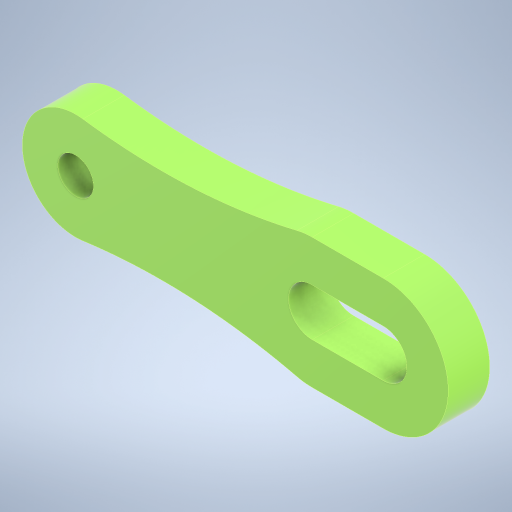
# Autodesk Inventor part: Elbow holder
Saved by Autodesk Inventor 2023 (Build 270158000, 158)
## iProperties
Created: 2022-05-02
Part Number: Elbow holder
Material: Phenolic Resin
Document SubType Name: Modeling
Designer: Devin
Density: 1.38 g/cm^3
Appearance: Light Green
Author: Devin
Autodesk Inventor part; units mm, degrees
ref_plane "YZ Plane" through (0, 0, 0) normal (1, 0, 0) x (0, 1, 0)
ref_plane "XZ Plane" through (0, 0, 0) normal (0, 1, 0) x (-1, 0, 0)
ref_plane "XY Plane" through (0, 0, 0) normal (0, 0, 1) x (1, 0, 0)
sketch "Sketch1" plane through (0, 0, 0) normal (0, 0, 1) x (1, 0, 0)
  line L0 (1.016, 0) -> (4.064, 0)
  line L1 (5.08, -1.016) -> (5.08, -1.016)
  line L2 (4.064, -2.032) -> (1.016, -2.032)
  line L3 (0, -1.016) -> (0, -1.016)
  line L4 (1.016, -3.81) -> (4.064, -3.81)
  line L5 (6.858, -1.016) -> (6.858, -1.016)
  line L6 (4.064, 1.778) -> (1.016, 1.778)
  line L7 (-1.778, -1.016) -> (-1.778, -1.016)
  arc A0 (6.858, -1.016) -> (4.064, 1.778) centre (4.064, -1.016) ccw
  arc A1 (4.064, -3.81) -> (6.858, -1.016) centre (4.064, -1.016) ccw
  arc A2 (5.08, -1.016) -> (4.064, 0) centre (4.064, -1.016) ccw
  arc A3 (4.064, -2.032) -> (5.08, -1.016) centre (4.064, -1.016) ccw
  arc A4 (1.016, 0) -> (0, -1.016) centre (1.016, -1.016) ccw
  arc A5 (0, -1.016) -> (1.016, -2.032) centre (1.016, -1.016) ccw
  circle A6 centre (-9.144, -1.016) radius 2.286
  circle A7 centre (-9.144, -1.016) radius 0.762
  arc A8 (1.016, 1.778) -> (-1.778, -1.016) centre (1.016, -1.016) ccw
  arc A9 (-1.778, -1.016) -> (1.016, -3.81) centre (1.016, -1.016) ccw
  arc A10 (-8.8323, 1.2486) -> (0.3651, 1.7011) centre (-5.4362, 25.9197) ccw
  arc A11 (0.3651, -3.7331) -> (-8.8323, -3.2806) centre (-5.4362, -27.9517) ccw
  line L8 (-8.0967, 1.016) -> (-0.9017, 1.016) construction
  line L9 (-8.0967, -3.048) -> (-0.9017, -3.048) construction
  line L10 (-6.858, -1.016) -> (-1.778, -1.016) construction
  point P0 (0, 0)
  point P1 (5.08, -2.032)
  point P2 (5.08, 0)
  point P3 (0, -2.032)
  point P4 (6.858, -3.81)
  point P5 (6.858, 1.778)
  point P6 (-8.382, -1.016)
  point P7 (5.08, -1.016)
  dimension "d15" = 1.524
  dimension "d0" = 5.08
  dimension "d1" = 2.032
  dimension "d2" = 1.778
  dimension "d3" = 5.588
  dimension "d4" = 2.794
  dimension "d5" = 2.794
  dimension "d6" = 1.016
  dimension "d8" = 1.524
  dimension "d9" = 2.794
  dimension "d10" = 8.382
  dimension "d11" = 4.064
  dimension "d12" = 2.032
  constraints: 29 point on circle, 22 end point, 22 tangent, 12 point on line, 11 centre point, 5 parallel, 4 equal radius, 3 horizontal, 2 horizontal alignment, 2 perpendicular, 1 coincident, 5 other
  measures "d0" distance of point (5.08, -2.032) point (0, -2.032)
  measures "d1" distance of point (5.08, 0) point (5.08, -2.032)
  measures "d2" distance between parallel lines of L2 L4
  measures "d3" distance of point (6.858, -3.81) point (6.858, 1.778)
  measures "d4" radius of A0
  measures "d5" radius of A1
  measures "d6" radius of A2
  measures "d9" radius of A8
  measures "d10" distance of point (-8.382, -1.016) point (0, -1.016)
  measures "d11" distance between parallel lines of L8 L9
  measures "d12" distance between parallel lines of L8 L10
extrude "Extrusion1" add sketch "Sketch1" along normal blind 1.778
body "Solid1"
